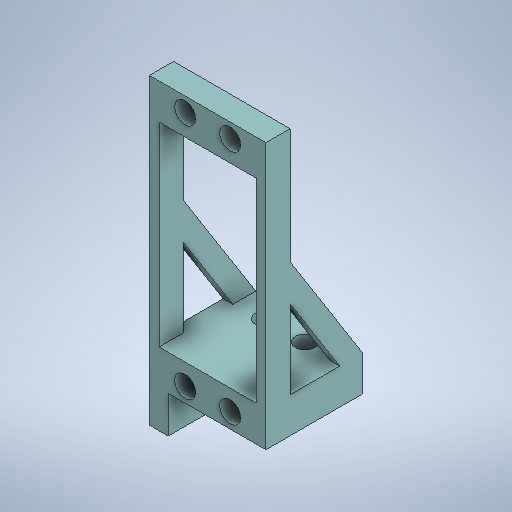
# Autodesk Inventor part: BIGServoHolder
Saved by Autodesk Inventor 2025.1 (Build 291241000, 241)
## iProperties
Created: 2025-02-24
Part Number: BIGServoHolder
Material: Generic
Document SubType Name: Modeling
Designer: 13156
Density: 1 g/cm^3
Appearance: Default
Author: 13156
Autodesk Inventor part; units mm, degrees
ref_plane "YZ Plane" through (0, 0, 0) normal (1, 0, 0) x (0, 1, 0)
ref_plane "XZ Plane" through (0, 0, 0) normal (0, 1, 0) x (-1, 0, 0)
ref_plane "XY Plane" through (0, 0, 0) normal (0, 0, 1) x (1, 0, 0)
sketch "Sketch1" plane through (0, 0, 0) normal (0, 0, 1) x (1, 0, 0)
  line L0 (-12.05, 27.5) -> (12.05, 27.5)
  line L1 (12.05, 27.5) -> (12.05, -27.5)
  line L2 (12.05, -27.5) -> (-12.05, -27.5)
  line L3 (-12.05, -27.5) -> (-12.05, 27.5)
  line L4 (-10.05, 20.15) -> (10.05, 20.15)
  line L5 (10.05, 20.15) -> (10.05, -20.15)
  line L6 (10.05, -20.15) -> (-10.05, -20.15)
  line L7 (-10.05, -20.15) -> (-10.05, 20.15)
  line L8 (0, 0) -> (0, 17.7516) construction
  line L9 (0, 0) -> (17.0454, 0) construction
  line L10 (-12.05, -27.5) -> (12.05, -27.5)
  line L11 (12.05, -27.5) -> (12.05, -20.15)
  line L12 (12.05, -20.15) -> (-12.05, -20.15)
  line L13 (-12.05, -20.15) -> (-12.05, -27.5)
  circle A0 centre (-4.65, 24.5) radius 2.175
  circle A1 centre (4.65, 24.475) radius 2.175
  circle A2 centre (-4.6492, -24.5) radius 2.175
  circle A3 centre (4.65, -24.375) radius 2.175
  point P0 (12.05, -23.825)
  dimension "d0" = 40.3
  dimension "d1" = 20.1
  dimension "d2" = 55
  dimension "d3" = 24.1
  dimension "d4" = 4.35
  dimension "d5" = 4.325
  dimension "d6" = 4.35
  dimension "d8" = 4.35
  dimension "d9" = 5.4
  dimension "d13" = 5.4
  dimension "d28" = 48.85
  dimension "d29" = 9.3
  dimension "d30" = 9.3
  constraints: 28 end point, 6 parallel, 4 centre point, 4 horizontal, 3 equal radius, 3 perpendicular, 1 collinear, 1 midpoint, 1 point on line, 1 vertical, 4 other
  measures "d0" distance between parallel lines of L6 L4
  measures "d1" distance between parallel lines of L5 L7
  measures "d2" distance between parallel lines of L2 L0
  measures "d3" distance between parallel lines of L1 L3
  measures "d4" diameter of A1
  measures "d5" distance from line of L4 A1.centre
  measures "d6" distance from line of L4 A0.centre
  measures "d8" distance from line of L6 A2.centre
  measures "d9" distance from line of L5 A1.centre
  measures "d13" distance from line of L5 A3.centre
  measures "d28" distance of A1.centre A3.centre
  measures "d29" distance of A2.centre A3.centre
  measures "d30" distance of A1.centre A0.centre
extrude "Extrusion1" add sketch "Sketch1" along normal blind 5 contours L0 L1 L12 L5 L4 L7 L3 | L12 L6 L1 L2 L3
extrude "Extrusion2" add sketch "Sketch1" against normal blind 15 contours L12 L6 L1 L2 L3 | A2 | A3
extrude "Extrusion3" cut sketch "Sketch1" against normal blind 3 contours A2 | A3
sketch "Sketch2" plane through (-10.05, -20.15, 5) normal (0, 1, 0) x (1, 0, 0)
  circle A0 centre (5.9, 16) radius 1.05
  circle A1 centre (14.2, 16) radius 1.05
  line L0 (0, 0) -> (20.1, 0) construction
  line L1 (10.05, 0) -> (10.05, 23.167) construction
  line L2 (-2, 20) -> (22.1, 20) projected
  circle A2 centre (14.2, 16) radius 2
  circle A3 centre (5.9, 16) radius 2
  point P0 (10.05, 5)
  dimension "d20" = 2.1
  dimension "d21" = 8.3
  dimension "d22" = 4
  dimension "d23" = 4
  constraints: 4 centre point, 2 coincident, 2 end point, 2 equal radius, 1 midpoint, 1 vertical, 1 other
  measures "d20" diameter of A0
  measures "d21" distance of A1.centre A0.centre
  measures "d22" distance from line of L2 A1.centre
  measures "d23" diameter of A2
extrude "Extrusion4" cut sketch "Sketch2" against normal blind 10 contours A0 | A1
extrude "Extrusion5" cut sketch "Sketch2" against normal blind 3 contours A0 | A1 | A2 | A3
sketch "Sketch3" plane through (12.05, -20.15, 0) normal (1, 0, 0) x (0, 0, -1)
  line L0 (-12.1039, 23.825) -> (31.505, 23.825) construction
  line L1 (0, 47.65) -> (-5, 47.65) construction
  line L2 (-5, 47.65) -> (38.6712, 47.65) construction
  line L3 (0, 0) -> (-5, 0) construction
  line L4 (-5, 0) -> (38.6712, 0) construction
  line L5 (-0.0214, 23.825) -> (15, 0)
  line L6 (-0.0214, 23.825) -> (-0.0214, 16.325)
  line L7 (-0.0214, 16.325) -> (10.2713, 0)
  line L8 (10.2713, 0) -> (15, 0)
  line L9 (15, 0) -> (15, -7.35) construction
  line L10 (15, -0.9137) -> (15, 2.4866) construction
  line L11 (-5, 0) -> (15, 0)
  line L12 (15, 0) -> (15, -15)
  line L13 (15, -15) -> (-5, -15)
  line L14 (-5, -15) -> (-5, 0)
  circle A0 centre (5, -10) radius 1.05
  point P0 (0, 20.15)
  dimension "d31" = 4
  dimension "d32" = 7.5
  dimension "d34" = 15
  dimension "d39" = 2.1
  dimension "d40" = 10
  dimension "d41" = 10
  constraints: 24 end point, 4 horizontal, 3 parallel, 3 point on line, 2 collinear, 1 centre point, 1 perpendicular, 1 vertical, 1 other
  measures "d31" distance between parallel lines of L7 L5
  measures "d32" distance of L5.start L6.end
  measures "d34" distance between parallel lines of L4 L13
  measures "d39" diameter of A0
  measures "d40" distance from line of L4 A0.centre
  measures "d41" distance from line of L12 A0.centre
ref_plane "Work Plane1" through (0, -20.15, 0) normal (-1, 0, 0) x (0, 0, 1)
extrude "Extrusion6" add sketch "Sketch3" against normal up to surface (2 mm away) contours L5 L8 L7 L6
mirror "Mirror1" about plane through (0, -20.15, 0) normal (-1, 0, 0) of "Extrusion6"
extrude "Extrusion7" add sketch "Sketch3" along normal blind 3.9 from surface at -24.1 contours L12 L13 L14 L11 L8 | A0
extrude "Extrusion8" cut sketch "Sketch3" against normal blind 35.65 contours A0
equation "\"d8\" = d6"
equation "\"d13\" = d9"
body "Solid1"
